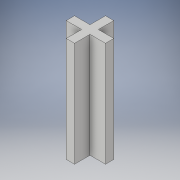
# Autodesk Inventor part: Brazo_union
Saved by Autodesk Inventor 2019 (Build 230136000, 136)
## iProperties
Created: 2020-02-09
Part Number: Brazo_union
Material: Generic
Document SubType Name: Modeling
Designer: Omar
Density: 1 g/cm^3
Appearance: Default
Author: Omar
Autodesk Inventor part; units mm, degrees
ref_plane "YZ Plane" through (0, 0, 0) normal (1, 0, 0) x (0, 1, 0)
ref_plane "XZ Plane" through (0, 0, 0) normal (0, 1, 0) x (-1, 0, 0)
ref_plane "XY Plane" through (0, 0, 0) normal (0, 0, 1) x (1, 0, 0)
sketch "Sketch1" plane through (0, 0, 0) normal (0, 1, 0) x (-1, 0, 0)
  line L0 (-7.5, 1.59) -> (7.5, 1.59)
  line L1 (7.5, 1.59) -> (7.5, -1.59)
  line L2 (7.5, -1.59) -> (-7.5, -1.59)
  line L3 (-7.5, -1.59) -> (-7.5, 1.59)
  line L4 (-7.5, 1.59) -> (7.5, -1.59) construction
  line L5 (7.5, 1.59) -> (-7.5, -1.59) construction
  line L6 (-1.59, 7.5) -> (1.59, 7.5)
  line L7 (1.59, 7.5) -> (1.59, -7.5)
  line L8 (1.59, -7.5) -> (-1.59, -7.5)
  line L9 (-1.59, -7.5) -> (-1.59, 7.5)
  line L10 (-1.59, 7.5) -> (1.59, -7.5) construction
  line L11 (1.59, 7.5) -> (-1.59, -7.5) construction
  point P0 (0, 0)
  dimension "d0" = 15
  dimension "d1" = 3.18
  dimension "d2" = 3.18
  dimension "d3" = 15
  constraints: 24 end point, 4 midpoint, 4 parallel, 2 horizontal, 2 perpendicular
  measures "d0" distance of L1.end L2.end
  measures "d1" distance of L0.end L1.end
  measures "d2" distance of L7.end L8.end
  measures "d3" distance of L6.end L7.end
extrude "Extrusion1" add sketch "Sketch1" along normal blind 40
body "Solid1"
